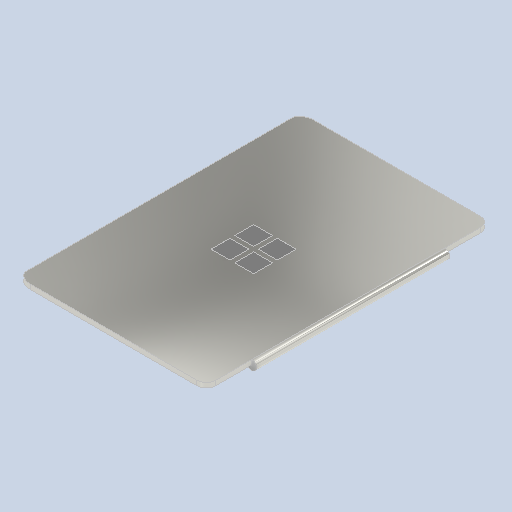
# Autodesk Inventor part: LaptopScreen
Saved by Autodesk Inventor 2022 (Build 260153000, 153)
## iProperties
Created: 2023-01-02
Part Number: LaptopScreen
Material: Generic
Document SubType Name: Modeling
Designer: mihir
Density: 1 g/cm^3
Appearance: Anodized - Black
Author: mihir
Autodesk Inventor part; units mm, degrees
ref_plane "YZ Plane" through (0, 0, 0) normal (1, 0, 0) x (0, 1, 0)
ref_plane "XZ Plane" through (0, 0, 0) normal (0, 1, 0) x (-1, 0, 0)
ref_plane "XY Plane" through (0, 0, 0) normal (0, 0, 1) x (1, 0, 0)
ref_plane "Work Plane1" through (0, 0.5, 0) normal (0, 1, 0) x (1, 0, 0)
sketch "Sketch2" plane through (0, 0.5, 0) normal (0, 1, 0) x (1, 0, 0)
  line L0 (18.5858, -4.8) -> (18.5858, -1)
  line L1 (17.5858, 0) -> (0, 0)
  line L2 (-1.4142, -1) -> (-1.4142, -29)
  line L3 (0, -30) -> (17.5858, -30)
  line L4 (18.5858, -25.2) -> (18.5858, -29)
  line L5 (18.5858, -25.2) -> (17.5858, -25.2)
  line L6 (17.5858, -4.8) -> (18.5858, -4.8)
  arc A0 (18.5858, -1) -> (17.5858, 0) centre (17.5858, -1) ccw
  line L7 (17.5858, -4.8) -> (17.5858, -25.2)
  arc A1 (17.5858, -30) -> (18.5858, -29) centre (17.5858, -29) ccw
  ellipse E0 centre (0, -29) end of major axis (-1.4142, -29) minor radius 1 (-1.4142, -29) -> (0, -30) ccw
  ellipse E1 centre (0, -1) end of major axis (-1.4142, -1) minor radius 1 (0, 0) -> (-1.4142, -1) ccw
  line L8 (16.9668, -0.619) -> (0, -0.619)
  line L9 (-0.7952, -1) -> (-0.7952, -29)
  line L10 (0, -29.381) -> (16.9668, -29.381)
  line L11 (16.9668, -25.819) -> (16.9668, -4.181)
  line L12 (16.9668, -25.819) -> (16.9668, -29.381)
  line L13 (16.9668, -4.181) -> (16.9668, -0.619)
  line L14 (0, -29.381) -> (-0.7952, -29.381)
  line L15 (-0.7952, -29.381) -> (-0.7952, -29)
  line L16 (-0.7952, -1) -> (-0.7952, -0.619)
  line L17 (-0.7952, -0.619) -> (0, -0.619)
  point P0 (17.5858, -25.819)
  constraints: 36 end point, 4 horizontal, 4 point on circle, 3 perpendicular, 2 centre point, 2 point on line, 2 vertical, 9 other
extrude "Extrusion2" add sketch "Sketch2" against normal blind 0.5
extrude "Extrusion3" add sketch "Sketch2" against normal blind 0.49 contours L13 L11 L12 L10 L14 L15 L9 L16 L17 L8
sketch "Sketch3" plane through (0, 0.5, 0) normal (0, 1, 0) x (1, 0, 0)
  line L0 (6.3358, -17.25) -> (8.3358, -17.25)
  line L1 (8.3358, -17.25) -> (8.3358, -15.25)
  line L2 (8.3358, -15.25) -> (6.3358, -15.25)
  line L3 (6.3358, -15.25) -> (6.3358, -17.25)
  line L4 (6.3358, -14.75) -> (8.3358, -14.75)
  line L5 (8.3358, -14.75) -> (8.3358, -12.75)
  line L6 (8.3358, -12.75) -> (6.3358, -12.75)
  line L7 (6.3358, -12.75) -> (6.3358, -14.75)
  line L8 (8.8358, -17.25) -> (10.8358, -17.25)
  line L9 (10.8358, -17.25) -> (10.8358, -15.25)
  line L10 (10.8358, -15.25) -> (8.8358, -15.25)
  line L11 (8.8358, -15.25) -> (8.8358, -17.25)
  line L12 (8.8358, -14.75) -> (10.8358, -14.75)
  line L13 (10.8358, -14.75) -> (10.8358, -12.75)
  line L14 (10.8358, -12.75) -> (8.8358, -12.75)
  line L15 (8.8358, -12.75) -> (8.8358, -14.75)
  line L16 (0, -30) -> (17.5858, -30) projected
  line L17 (18.5858, -4.8) -> (18.5858, -1) projected
  point P0 (0, 0)
  dimension "d11" = 2
  dimension "d12" = 2
  dimension "d13" = 0.5
  dimension "d14" = 0.5
  dimension "d15" = 0.5
  dimension "d16" = 12.75
  dimension "d17" = 7.75
  constraints: 32 end point, 8 parallel, 5 equal length, 4 horizontal, 4 perpendicular, 4 point on line
  measures "d11" distance of L0.start L0.end
  measures "d12" distance of L2.end L0.start
  measures "d13" distance between parallel lines of L1 L11
  measures "d14" distance between parallel lines of L12 L10
  measures "d15" distance between parallel lines of L2 L4
  measures "d16" distance between parallel lines of L16 L8
  measures "d17" distance between parallel lines of L17 L13
extrude "Extrusion4" add sketch "Sketch3" along normal blind 0.001
sketch "Sketch4" plane through (0, 0, 0) normal (0, -1, 0) x (1, 0, 0)
  circle A0 centre (-1.1102, 15) radius 0.125
  line L0 (-0.7952, 0.619) -> (-0.7952, 29.381) projected
  line L1 (0, 0) -> (17.5858, 0) projected
  dimension "d20" = 0.25
  dimension "d21" = 0.315
  dimension "d22" = 15
  constraints: 1 centre point
  measures "d20" diameter of A0
  measures "d21" distance from line of L0 A0.centre
  measures "d22" distance from line of A0.centre L1
extrude "Extrusion5" add sketch "Sketch4" along normal blind 0.001
sketch "Sketch5" plane through (18.5858, 0.5, 25.2) normal (0, 0, -1) x (-1, 0, 0)
  line L0 (0.25, -0.275) -> (0.25, -0.5)
  line L1 (0.75, -0.5) -> (0.75, -0.275)
  arc A0 (0.75, -0.275) -> (0.25, -0.275) centre (0.5, -0.275) ccw
  line L2 (1, 0) -> (1, -0.5) projected
  line L3 (0, 0) -> (1, 0) projected
  line L4 (1, -0.5) -> (0, -0.5) projected
  line L5 (0, -0.5) -> (1, -0.5) projected
  arc A1 (0.5, 0) -> (0, -0.5) centre (0.5, -0.5) ccw
  line L6 (0, 0) -> (0, -0.5) projected
  circle A2 centre (0, -0.5) radius 0.5
  point P0 (18.5858, -0.5)
  point P1 (0.5, -0.975)
  point P2 (0.75, -0.5)
  point P3 (0.25, -0.5)
  point P4 (0.5, -0.5)
  dimension "d26" = 0
  dimension "d36" = 0.5
  constraints: 5 end point, 5 point on circle, 3 point on line, 2 centre point, 2 coincident, 2 tangent, 1 midpoint, 1 parallel, 3 other
  measures "d26" horizontal distance of point (0.5, -0.5) A0.centre
  measures "d36" distance from line of L6 point (0.5, -0.5)
sketch "Sketch6" plane through (18.5858, 0.5, 25.2) normal (0, 0, -1) x (-1, 0, 0)
  line L0 (1, 0) -> (1, -0.5) projected
  line L1 (0, 0) -> (1, 0) projected
  line L2 (1, -0.5) -> (0, -0.5)
  line L3 (0, -0.5) -> (0, 0)
  line L4 (0, 0) -> (1, 0)
  line L5 (1, 0) -> (1, -0.5)
  point P0 (18.5858, -0.5)
  constraints: 8 end point, 2 parallel, 1 horizontal, 1 perpendicular
extrude "Extrusion6" add sketch "Sketch6" along normal blind 21.5
extrude "Extrusion7" add sketch "Sketch5" along normal blind 20.425 contours A0 A2 L4 L0 | L4 A2 L6 | A0 L1 L4 A2
body "Solid2"
